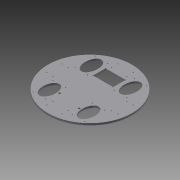
# Autodesk Inventor part: Base_Acryllic
Saved by Autodesk Inventor 2015 SP1 (Build 190203100, 203)
## iProperties
Created: 2016-03-29
Part Number: Base_Acryllic
Material: Generic
Document SubType Name: Modeling
Designer: Ethan
Density: 1 g/cm^3
Appearance: Default
Author: Ethan
Autodesk Inventor part; units mm, degrees
ref_plane "YZ Plane" through (0, 0, 0) normal (1, 0, 0) x (0, 1, 0)
ref_plane "XZ Plane" through (0, 0, 0) normal (0, 1, 0) x (-1, 0, 0)
ref_plane "XY Plane" through (0, 0, 0) normal (0, 0, 1) x (1, 0, 0)
sketch "Sketch1" plane through (0, 0, 0) normal (0, 1, 0) x (-1, 0, 0)
  circle A0 centre (0, 0) radius 139.7
  circle A1 centre (-118.5333, 25.4) radius 1.5875
  circle A2 centre (-97.3667, 25.4) radius 1.5875
  circle A3 centre (-118.5333, -25.4) radius 1.5875
  circle A4 centre (-97.3667, -25.4) radius 1.5875
  line L0 (33.3375, -43.706) -> (-33.3375, -43.706)
  line L1 (-33.3375, -43.706) -> (-33.3375, -84.981)
  line L2 (-33.3375, -84.981) -> (33.3375, -84.981)
  line L3 (33.3375, -84.981) -> (33.3375, -43.706)
  ellipse E0 centre (-65.0875, 69.8532) end of major axis (-65.0875, 36.5157) minor radius 20.6375
  ellipse E1 centre (-65.0875, -69.8532) end of major axis (-65.0875, -36.5157) minor radius 20.6375
  ellipse E2 centre (65.0875, 69.8532) end of major axis (65.0875, 36.5157) minor radius 20.6375
  ellipse E3 centre (65.0875, -69.8532) end of major axis (65.0875, -36.5157) minor radius 20.6375
  circle A5 centre (-38.1, 74.0494) radius 3.175
  circle A6 centre (38.1, 62.9369) radius 3.175
  circle A7 centre (85.725, 103.1907) radius 1.5875
  circle A8 centre (44.45, 103.1907) radius 1.5875
  circle A9 centre (85.725, 36.5157) radius 1.5875
  circle A10 centre (44.45, 36.5157) radius 1.5875
  circle A11 centre (44.45, -36.5157) radius 1.5875
  circle A12 centre (44.45, -103.1907) radius 1.5875
  circle A13 centre (85.725, -103.1907) radius 1.5875
  circle A14 centre (85.725, -36.5157) radius 1.5875
  circle A15 centre (33.3375, -43.706) radius 1.5875
  circle A16 centre (33.3375, -84.981) radius 1.5875
  circle A17 centre (-33.3375, -84.981) radius 1.5875
  circle A18 centre (-33.3375, -43.706) radius 1.5875
  circle A19 centre (-44.45, 36.5157) radius 1.5875
  circle A20 centre (-44.45, 103.1907) radius 1.5875
  circle A21 centre (-85.725, 103.1907) radius 1.5875
  circle A22 centre (-85.725, 36.5157) radius 1.5875
  circle A23 centre (-85.725, -36.5157) radius 1.5875
  circle A24 centre (-44.45, -36.5157) radius 1.5875
  circle A25 centre (-44.45, -103.1907) radius 1.5875
  circle A26 centre (-85.725, -103.1907) radius 1.5875
  circle A27 centre (-25.4, -118.5333) radius 1.5875
  circle A28 centre (-25.4, -97.3667) radius 1.5875
  circle A29 centre (25.4, -97.3667) radius 1.5875
  circle A30 centre (25.4, -118.5333) radius 1.5875
  circle A31 centre (118.5333, -25.4) radius 1.5875
  circle A32 centre (97.3667, -25.4) radius 1.5875
  circle A33 centre (97.3667, 25.4) radius 1.5875
  circle A34 centre (118.5333, 25.4) radius 1.5875
  circle A35 centre (25.4, 118.5333) radius 1.5875
  circle A36 centre (25.4, 97.3667) radius 1.5875
  circle A37 centre (-25.4, 97.3667) radius 1.5875
  circle A38 centre (-25.4, 118.5333) radius 1.5875
  dimension "d0" = 279.4
  dimension "d1" = 3.175
  dimension "d4" = 3.175
  dimension "d5" = 21.1667
  dimension "d22" = 66.675
  dimension "d23" = 41.275
  dimension "d29" = 6.35
  dimension "d30" = 6.35
  dimension "d31" = 11.1125
  dimension "d32" = 3.175
  dimension "d33" = 3.175
  dimension "d34" = 3.175
  dimension "d35" = 3.175
  dimension "d36" = 3.175
  dimension "d37" = 3.175
  dimension "d38" = 3.175
  dimension "d39" = 3.175
  dimension "d40" = 3.175
  dimension "d41" = 3.175
  dimension "d42" = 3.175
  dimension "d43" = 3.175
  dimension "d44" = 3.175
  dimension "d45" = 3.175
  dimension "d46" = 3.175
  dimension "d47" = 3.175
  dimension "d48" = 3.175
  dimension "d49" = 3.175
  dimension "d50" = 3.175
  dimension "d51" = 3.175
  dimension "d56" = 360
  constraints: 39 centre point, 8 end point, 2 parallel, 1 coincident, 1 horizontal, 1 perpendicular, 41 other
  measures "d0" diameter of A0
  measures "d1" diameter of A1
  measures "d4" diameter of A2
  measures "d5" distance of A1.centre A2.centre
  measures "d22" distance of L1.end L2.end
  measures "d23" distance of L0.end L1.end
  measures "d29" diameter of A5
  measures "d30" diameter of A6
  measures "d31" vertical distance of A6.centre A5.centre
  measures "d32" diameter of A7
  measures "d33" diameter of A8
  measures "d34" diameter of A9
  measures "d35" diameter of A10
  measures "d36" diameter of A11
  measures "d37" diameter of A12
  measures "d38" diameter of A13
  measures "d39" diameter of A14
  measures "d40" diameter of A15
  measures "d41" diameter of A16
  measures "d42" diameter of A17
  measures "d43" diameter of A18
  measures "d44" diameter of A19
  measures "d45" diameter of A20
  measures "d46" diameter of A21
  measures "d47" diameter of A22
  measures "d48" diameter of A23
  measures "d49" diameter of A24
  measures "d50" diameter of A25
  measures "d51" diameter of A26
extrude "Extrusion2" add sketch "Sketch1" along normal blind 6.35
body "Solid2"
